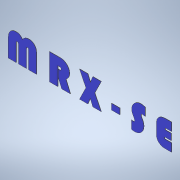
# Autodesk Inventor part: Logo
Saved by Autodesk Inventor 2021.2 (Build 252289000, 289)
## iProperties
Created: 2026-06-08
Part Number: Logo
Material: Generic
Document SubType Name: Modeling
Designer: NELSON
Density: 1 g/cm^3
Appearance: Default
Author: NELSON
Autodesk Inventor part; units mm, degrees
ref_plane "YZ Plane" through (0, 0, 0) normal (1, 0, 0) x (0, 1, 0)
ref_plane "XZ Plane" through (0, 0, 0) normal (0, 1, 0) x (-1, 0, 0)
ref_plane "XY Plane" through (0, 0, 0) normal (0, 0, 1) x (1, 0, 0)
sketch "Boceto1" plane through (0, 0, 0) normal (0, 0, 1) x (1, 0, 0)
  line L0 (-10.159, 4.8662) -> (417.1829, 4.8662) construction
  line L1 (417.1829, 4.8662) -> (417.1829, -72.825) construction
  line L2 (417.1829, -72.825) -> (-10.159, -72.825) construction
  line L3 (-10.159, -72.825) -> (-10.159, 4.8662) construction
  line L4 (34.6033, -50.1338) -> (34.6033, -15.4319)
  spline S0 degree 2 poles (34.6033, -15.4319) (34.6033, -12.9057) (33.584, -11.3989) (32.343, -11.3989) knots 0 0 0 1 2 2 2
  spline S1 degree 2 poles (32.343, -11.3989) (30.9691, -11.3989) (29.8612, -12.95) (29.8612, -15.4319) knots 0 0 0 1 2 2 2
  line L5 (29.8612, -15.4319) -> (29.8612, -50.1338)
  line L6 (29.8612, -50.1338) -> (13.4631, -50.1338)
  line L7 (13.4631, -50.1338) -> (13.4631, -15.4319)
  spline S2 degree 2 poles (13.4631, -15.4319) (13.4631, -12.9057) (12.4438, -11.3989) (11.2028, -11.3989) knots 0 0 0 1 2 2 2
  spline S3 degree 2 poles (11.2028, -11.3989) (9.8289, -11.3989) (8.721, -12.95) (8.721, -15.4319) knots 0 0 0 1 2 2 2
  line L8 (8.721, -15.4319) -> (8.721, -50.1338)
  line L9 (8.721, -50.1338) -> (-7.4998, -50.1338)
  line L10 (-7.4998, -50.1338) -> (-7.4998, -15.7865)
  spline S4 degree 2 poles (-7.4998, -15.7865) (-7.4998, -10.3795) (-6.3919, -4.7067) (-5.0623, -2.4907) knots 0 0 0 1 2 2 2
  spline S5 degree 2 poles (-5.0623, -2.4907) (-2.935, 1.0548) (4.1118, 4.8662) (8.4994, 4.8662) knots 0 0 0 1 2 2 2
  spline S6 degree 2 poles (8.4994, 4.8662) (12.887, 4.8662) (20.0223, 0.7002) (21.6621, -2.7567) knots 0 0 0 1 2 2 2
  spline S7 degree 2 poles (21.6621, -2.7567) (23.3463, 0.7446) (30.393, 4.8662) (34.7806, 4.8662) knots 0 0 0 1 2 2 2
  spline S8 degree 2 poles (34.7806, 4.8662) (38.6363, 4.8662) (45.0626, 1.9855) (47.2343, -0.8066) knots 0 0 0 1 2 2 2
  spline S9 degree 2 poles (47.2343, -0.8066) (49.1843, -3.1998) (50.8684, -9.5818) (50.8684, -15.7865) knots 0 0 0 1 2 2 2
  line L11 (50.8684, -15.7865) -> (50.8684, -50.1338)
  line L12 (50.8684, -50.1338) -> (34.6033, -50.1338)
  line L13 (95.7193, -18.357) -> (98.1569, -18.357)
  spline S10 degree 2 poles (98.1569, -18.357) (100.1956, -18.357) (101.7024, -17.0274) (101.7024, -15.3876) knots 0 0 0 1 2 2 2
  spline S11 degree 2 poles (101.7024, -15.3876) (101.7024, -13.8364) (100.3729, -12.6841) (98.1569, -12.6841) knots 0 0 0 1 2 2 2
  line L14 (98.1569, -12.6841) -> (94.7886, -12.6841)
  line L15 (94.7886, -12.6841) -> (94.7886, -50.1338)
  line L16 (94.7886, -50.1338) -> (77.5928, -50.1338)
  line L17 (77.5928, -50.1338) -> (77.5928, 3.8026)
  line L18 (77.5928, 3.8026) -> (97.5807, 3.8026)
  spline S12 degree 2 poles (97.5807, 3.8026) (103.0763, 3.8026) (108.9264, 2.0298) (111.6299, 0.0798) knots 0 0 0 1 2 2 2
  spline S13 degree 2 poles (111.6299, 0.0798) (115.2197, -2.5794) (119.1198, -10.2909) (119.1198, -14.6342) knots 0 0 0 1 2 2 2
  spline S14 degree 2 poles (119.1198, -14.6342) (119.1198, -18.8445) (115.3527, -25.8026) (111.7629, -28.4617) knots 0 0 0 1 2 2 2
  line L19 (111.7629, -28.4617) -> (120.8926, -50.1338)
  line L20 (120.8926, -50.1338) -> (103.1206, -50.1338)
  line L21 (103.1206, -50.1338) -> (95.7193, -33.0709)
  line L22 (95.7193, -33.0709) -> (95.7193, -18.357)
  line L23 (139.8168, 3.8026) -> (157.0127, 3.8026)
  line L24 (157.0127, 3.8026) -> (162.198, -8.7397)
  line L25 (162.198, -8.7397) -> (167.2504, 3.8026)
  line L26 (167.2504, 3.8026) -> (184.5791, 3.8026)
  line L27 (184.5791, 3.8026) -> (171.2391, -23.1878)
  line L28 (171.2391, -23.1878) -> (184.5791, -50.1338)
  line L29 (184.5791, -50.1338) -> (167.2947, -50.1338)
  line L30 (167.2947, -50.1338) -> (162.198, -37.5471)
  line L31 (162.198, -37.5471) -> (157.0127, -50.1338)
  line L32 (157.0127, -50.1338) -> (139.8168, -50.1338)
  line L33 (139.8168, -50.1338) -> (153.0683, -23.1878)
  line L34 (153.0683, -23.1878) -> (139.8168, 3.8026)
  line L35 (205.9853, -36.5278) -> (205.9853, -24.473)
  line L36 (205.9853, -24.473) -> (223.1811, -24.473)
  line L37 (223.1811, -24.473) -> (223.1811, -36.5278)
  line L38 (223.1811, -36.5278) -> (205.9853, -36.5278)
  line L39 (246.9804, -50.0895) -> (246.9804, -33.8687)
  spline S15 degree 2 poles (246.9804, -33.8687) (248.9748, -34.1346) (250.1271, -34.2675) (250.6146, -34.2675) knots 0 0 0 1 2 2 2
  spline S16 degree 2 poles (250.6146, -34.2675) (252.2101, -34.2675) (253.9828, -32.5834) (253.9828, -31.0766) knots 0 0 0 1 2 2 2
  spline S17 degree 2 poles (253.9828, -31.0766) (253.9828, -29.2595) (252.2101, -26.4231) knots 0 0 0 1 1 1
  spline S18 degree 2 poles (252.2101, -26.4231) (251.9885, -26.0685) (251.9442, -25.9355) knots 0 0 0 1 1 1
  line L40 (251.9442, -25.9355) -> (251.4567, -25.2264)
  spline S19 degree 2 poles (251.4567, -25.2264) (247.7782, -19.2434) (247.7782, -13.9694) knots 0 0 0 1 1 1
  spline S20 degree 2 poles (247.7782, -13.9694) (247.7782, -6.4351) (258.9023, 4.8662) (266.6581, 4.8662) knots 0 0 0 1 2 2 2
  spline S21 degree 2 poles (266.6581, 4.8662) (268.5195, 4.8662) (272.6412, 4.0242) (275.4333, 3.0048) knots 0 0 0 1 2 2 2
  line L41 (275.4333, 3.0048) -> (275.4333, -13.3932)
  spline S22 degree 2 poles (275.4333, -13.3932) (273.0401, -12.7728) (271.09, -12.2853) (270.2923, -12.2853) knots 0 0 0 1 2 2 2
  spline S23 degree 2 poles (270.2923, -12.2853) (268.8741, -12.2853) (267.057, -14.058) (267.057, -15.5206) knots 0 0 0 1 2 2 2
  spline S24 degree 2 poles (267.057, -15.5206) (267.057, -16.9831) (268.7854, -19.8638) knots 0 0 0 1 1 1
  spline S25 degree 2 poles (268.7854, -19.8638) (269.14, -20.5286) (269.2286, -20.6616) knots 0 0 0 1 1 1
  spline S26 degree 2 poles (269.2286, -20.6616) (271.0457, -23.7196) (272.6855, -29.4368) (272.6855, -32.3175) knots 0 0 0 1 2 2 2
  spline S27 degree 2 poles (272.6855, -32.3175) (272.6855, -40.4279) (261.7387, -51.2417) (253.7612, -51.2417) knots 0 0 0 1 2 2 2
  spline S28 degree 2 poles (253.7612, -51.2417) (252.2987, -51.2417) (249.4623, -50.7986) (246.9804, -50.0895) knots 0 0 0 1 2 2 2
  line L42 (329.9015, -50.1338) -> (318.2455, -50.1338)
  spline S29 degree 2 poles (318.2455, -50.1338) (314.0795, -50.1338) (309.2044, -49.0701) (307.0328, -47.9178) knots 0 0 0 1 2 2 2
  spline S30 degree 2 poles (307.0328, -47.9178) (303.2214, -45.8348) (298.9667, -39.0983) (298.9667, -35.2426) knots 0 0 0 1 2 2 2
  line L43 (298.9667, -35.2426) -> (298.9667, -15.6092)
  spline S31 degree 2 poles (298.9667, -15.6092) (298.9667, -8.8727) (301.5372, -2.5794) (304.7282, -0.0089) knots 0 0 0 1 2 2 2
  spline S32 degree 2 poles (304.7282, -0.0089) (307.1214, 1.9855) (313.9466, 3.8026) (319.0876, 3.8026) knots 0 0 0 1 2 2 2
  line L44 (319.0876, 3.8026) -> (329.9015, 3.8026)
  line L45 (329.9015, 3.8026) -> (329.9015, -12.9944)
  line L46 (329.9015, -12.9944) -> (319.1762, -12.9944)
  spline S33 degree 2 poles (319.1762, -12.9944) (317.6694, -12.9944) (316.8273, -13.7035) (316.8273, -14.6342) knots 0 0 0 1 2 2 2
  spline S34 degree 2 poles (316.8273, -14.6342) (316.8273, -15.7422) (317.8023, -16.5842) (319.1762, -16.5842) knots 0 0 0 1 2 2 2
  line L47 (319.1762, -16.5842) -> (329.2367, -16.5842)
  line L48 (329.2367, -16.5842) -> (329.2367, -29.747)
  line L49 (329.2367, -29.747) -> (317.6694, -29.747)
  spline S35 degree 2 poles (317.6694, -29.747) (316.2512, -29.747) (315.4091, -30.4561) (315.4091, -31.3868) knots 0 0 0 1 2 2 2
  spline S36 degree 2 poles (315.4091, -31.3868) (315.4091, -32.5391) (316.3398, -33.3368) (317.6694, -33.3368) knots 0 0 0 1 2 2 2
  line L50 (317.6694, -33.3368) -> (329.9015, -33.3368)
  line L51 (329.9015, -33.3368) -> (329.9015, -50.1338)
  point P0 (0, 0)
  constraints: 2 other
extrude "Extrusión1" add sketch "Boceto1" along normal blind 0.6
